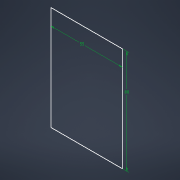
# Autodesk Inventor part: pcb main
Saved by Autodesk Inventor 2022 (Build 260153000, 153)
## iProperties
Created: 2021-08-27
Part Number: pcb main
Material: Ogólny
Document SubType Name: Modeling
Designer: Karol
Density: 1 g/cm^3
Appearance: Domyślna
Author: Karol
Autodesk Inventor part; units mm, degrees
ref_plane "YZ Plane" through (0, 0, 0) normal (1, 0, 0) x (0, 1, 0)
ref_plane "XZ Plane" through (0, 0, 0) normal (0, 1, 0) x (-1, 0, 0)
ref_plane "XY Plane" through (0, 0, 0) normal (0, 0, 1) x (1, 0, 0)
sketch "Szkic1" plane through (0, 0, 0) normal (0, 0, 1) x (1, 0, 0)
  line L0 (0, 0) -> (55, 0)
  line L1 (55, 0) -> (55, 65)
  line L2 (55, 65) -> (0, 65)
  line L3 (0, 65) -> (0, 0)
  dimension "d0" = 55
  dimension "d1" = 65
  constraints: 8 end point, 2 parallel, 1 horizontal, 1 perpendicular
  measures "d0" distance between parallel lines of L3 L1
  measures "d1" distance of L0.end L1.end
extrude "Wyciągnięcie proste1" add sketch "Szkic1" along normal blind 1.6
sketch "Szkic2" plane through (0, 0, 1.6) normal (0, 0, 1) x (1, 0, 0)
  circle A0 centre (50, 35) radius 0.6
  circle A1 centre (45, 35) radius 0.6
  circle A2 centre (40, 35) radius 0.6
  circle A3 centre (32.5, 20) radius 0.6
  circle A4 centre (27.5, 20) radius 0.6
  circle A5 centre (22.5, 20) radius 0.6
  circle A6 centre (15, 35) radius 0.6
  circle A7 centre (10, 35) radius 0.6
  circle A8 centre (5, 35) radius 0.6
  line L0 (55, 65) -> (0, 65) projected
  point P0 (0, 0)
  point P1 (27.5, 65)
  dimension "d4" = 15
  dimension "d5" = 5
  dimension "d6" = 5
  dimension "d7" = 5
  dimension "d8" = 5
  dimension "d9" = 5
  dimension "d10" = 5
  dimension "d11" = 30
  dimension "d12" = 17.5
  dimension "d13" = 17.5
  dimension "d14" = 1.2
  constraints: 9 centre point, 8 equal radius, 7 horizontal alignment, 1 midpoint, 1 vertical alignment
  measures "d4" vertical distance of A3.centre A2.centre
  measures "d5" distance of A1.centre A0.centre
  measures "d6" distance of A2.centre A1.centre
  measures "d7" distance of A4.centre A3.centre
  measures "d8" distance of A5.centre A4.centre
  measures "d9" distance of A7.centre A6.centre
  measures "d10" distance of A8.centre A7.centre
  measures "d11" distance from line of L0 A1.centre
  measures "d12" horizontal distance of A4.centre A1.centre
  measures "d13" horizontal distance of A4.centre A7.centre
  measures "d14" diameter of A0
extrude "Wyciągnięcie proste2" cut sketch "Szkic2" against normal blind 1.6
sketch "Szkic3" plane through (0, 0, 1.6) normal (0, 0, 1) x (1, 0, 0)
  circle A0 centre (27.5, 53.25) radius 4 projected
  point P0 (0, 0)
extrude "Wyciągnięcie proste3" cut sketch "Szkic3" against normal blind 1.6
equation "\"d6\" = d5"
equation "\"d7\" = d6"
equation "\"d8\" = d7"
equation "\"d9\" = d8"
equation "\"d10\" = d9"
equation "\"d13\" = d12"
